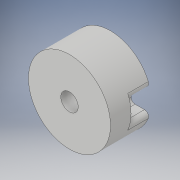
# Autodesk Inventor part: Tripod Mount
Saved by Autodesk Inventor 2019 (Build 230136000, 136)
## iProperties
Created: 2018-06-03
Part Number: Tripod Mount
Material: Generic
Document SubType Name: Modeling
Designer: samps
Density: 1 g/cm^3
Appearance: Default
Author: samps
Autodesk Inventor part; units mm, degrees
ref_plane "YZ Plane" through (0, 0, 0) normal (1, 0, 0) x (0, 1, 0)
ref_plane "XZ Plane" through (0, 0, 0) normal (0, 1, 0) x (-1, 0, 0)
ref_plane "XY Plane" through (0, 0, 0) normal (0, 0, 1) x (1, 0, 0)
sketch "Sketch1" plane through (0, 0, 0) normal (0, 0, 1) x (1, 0, 0)
  point P0 (0, 0)
sketch "Sketch2" plane through (0, 0, 0) normal (0, 0, 1) x (1, 0, 0)
  circle A0 centre (0, 0) radius 20
  dimension "d0" = 40
  constraints: 1 centre point, 1 coincident
  measures "d0" diameter of A0
extrude "Extrusion1" add sketch "Sketch2" along normal blind 20
sketch "Sketch3" plane through (0, 0, 20) normal (0, 0, 1) x (1, 0, 0)
  point P0 (0, 0)
  point P1 (0, 0)
  constraints: 1 coincident
hole "Hole1" at (0, 0, 20) direction (0, 0, -1) diameter 5.1 end through all
sketch "Sketch4" plane through (0, 0, 20) normal (0, 0, 1) x (1, 0, 0)
  point P0 (0, 0)
  point P1 (0, 0)
  constraints: 1 coincident
hole "Hole2" at (0, 0, 20) direction (0, 0, -1) diameter 8.5 depth 8 tip angle 118
sketch "Sketch5" plane through (0, 0, 0) normal (0, 0, -1) x (-1, 0, 0)
  line L0 (0, 0) -> (-10, 0)
  line L1 (-10, 0) -> (10, 0)
  line L2 (10, 0) -> (10, -5)
  line L3 (10, -5) -> (20, -5)
  line L4 (20, -5) -> (20, 5)
  line L5 (20, 5) -> (10, 5)
  line L6 (10, 5) -> (10, -5)
  line L7 (-10, -5) -> (-20, -5)
  line L8 (-20, -5) -> (-20, 5)
  line L9 (-20, 5) -> (-10, 5)
  line L10 (-10, 5) -> (-10, -5)
  dimension "d17" = 10
  dimension "d18" = 20
  dimension "d19" = 5
  dimension "d20" = 10
  dimension "d21" = 10
  constraints: 22 end point, 4 parallel, 3 horizontal, 2 perpendicular, 2 point on line, 1 vertical
  measures "d17" distance of L0.start L0.end
  measures "d18" distance of L0.end L1.end
  measures "d19" distance of L1.end L2.end
  measures "d20" distance of L4.end L3.end
  measures "d21" distance of L7.end L8.end
extrude "Extrusion2" cut sketch "Sketch5" against normal blind 10
sketch "Sketch6" plane through (10, -5, 0) normal (1, 0, 0) x (0, 0, -1)
  line L0 (0, 5) -> (-10, 5)
  line L1 (-10, 0) -> (-10, 10) projected
  point P0 (-5, 5)
  constraints: 2 end point, 2 midpoint
hole "Hole3" at (10, 0, 5) direction (-1, 0, 0) diameter 3.5 end through all
fillet "Fillet1" radius 2 8 edges at (10, 5, 5) (10, -5, 5) (19.3649, -5, 5) (19.3649, 5, 5) (-19.3649, 5, 5) (-19.3649, -5, 5) (-10, 5, 5) (-10, -5, 5)
body "Solid1"
